Autodesk Inventor part; units mm, degrees
(part 6 of 6)
extrude "Zifferblatt" cut sketch "Text" against normal blind 1 contours S0 L450 S1 S2 L451 L452 L453 S3 S4 L454 L455 L456 S5 S6 L457 S7 L458 | S8 S9 S10 S11 L459 L460 S12 S13 S14 S15 L461 S16 S17 L462 | S18 S19 L463 S20 S21 L464 | S22 S23 L465 S24 S25 L466 | S26 S27 S28 S29 S30 L467 S31 S32 L468 S33 S34 L469 S35 S36 L470 S37 S38 S39 S40 S41 S42 L471 S43 S44 L472 S45 S46 S47 S48 S49 L473 S50 | S51 S52 S53 S54 S55 L474 S56 S57 S58 S59 S60 S61 S62 L475 S63 S64 | S65 S66 L476 L477 L478 S67 S68 L479 S69 S70 L480 L481 L482 S71 S72 L483 | S73 S74 L484 L485 S75 S76 S77 S78 L486 S79 S80 S81 S82 L487 S83 S84 S85 S86 L488 L489 L490 | S87 S88 L491 L492 S89 S90 L493 S91 L494 S92 S93 L495 L496 L497 | S94 S95 L498 S96 S97 L499 S98 S99 L500 S100 S101 L501 | S102 S103 S104 S105 | S106 S107 S108 S109 | S110 S111 L502 L503 S112 S113 L504 S114 L505 S115 S116 L506 L507 L508 | S117 S118 S119 S120 L509 L510 S121 S122 S123 S124 L511 S125 S126 S127 S128 L512 | S129 S130 L513 S131 S132 L514 | S133 L515 S134 S135 L516 L517 L518 S136 S137 L519 L520 L521 S138 S139 L522 S140 L523 | S141 S142 L524 S143 L525 L526 S144 S145 L527 S146 L528 S147 L529 S148 S149 L530 S150 S151 S152 S153 S154 S155 L531 S156 S157 S158 | S159 S160 L532 S161 S162 L533 L534 S163 S164 L535 L536 | S165 S166 L537 S167 S168 L538 S169 S170 L539 S171 S172 L540 | S173 S174 S175 S176 S177 S178 S179 L541 S180 S181 S182 S183 L542 S184 S185 S186 S187 L543 S188 S189 S190 S191 S192 S193 S194 L544 S195 S196 L545 | S197 S198 L546 S199 S200 L547 | S201 S202 L548 L549 S203 S204 L550 S205 L551 S206 S207 L552 L553 L554 | S208 S209 L555 S210 S211 L556 L557 S212 S213 L558 S214 S215 L559 L560 | S216 S217 L561 L562 S218 S219 S220 S221 L563 S222 S223 S224 S225 L564 S226 S227 S228 S229 L565 L566 L567 | S230 S231 S232 S233 | S234 S235 S236 S237 | S238 S239 L568 L569 S240 S241 S242 S243 L570 S244 S245 S246 S247 L571 S248 S249 S250 S251 L572 L573 L574 | S252 S253 S254 S255 | S256 S257 S258 S259 | S260 S261 L575 S262 L576 L577 S263 S264 L578 S265 L579 S266 L580 S267 S268 L581 S269 S270 S271 S272 S273 S274 L582 S275 S276 S277 | S278 S279 S280 S281 S282 S283 L583 S284 S285 S286 S287 S288 S289 S290 S291 L584 S292 S293 | S294 S295 S296 S297 S298 S299 L585 S300 S301 S302 S303 S304 S305 S306 S307 L586 S308 S309 | S310 S311 S312 S313 L587 L588 S314 S315 S316 S317 L589 S318 S319 S320 S321 L590 | S322 S323 L591 S324 S325 L592 | S326 S327 S328 S329 S330 L593 S331 S332 L594 S333 S334 L595 S335 S336 L596 S337 S338 S339 S340 S341 S342 L597 S343 S344 L598 S345 S346 S347 S348 S349 L599 S350 | S351 S352 S353 S354 S355 L600 S356 L601 L602 L603 S357 S358 L604 S359 L605 S360 L606 S361 L607 S362 S363 | S364 S365 L608 S366 S367 L609 L610 S368 S369 L611 S370 S371 L612 L613 | S372 S373 L614 S374 S375 S376 L615 L616 S377 S378 L617 S379 S380 S381 S382 L618 L619 | S383 S384 L620 L621 S385 S386 S387 S388 L622 S389 S390 S391 S392 L623 S393 S394 S395 S396 L624 L625 L626 | S397 S398 S399 S400 | S401 S402 S403 S404 | S405 S406 S407 S408 L627 L628 S409 S410 S411 S412 L629 S413 S414 S415 S416 L630 L631 S417 S418 L632 L633 S419 S420 S421 S422 L634 | S423 S424 L635 S425 S426 L636 L637 S427 S428 L638 S429 S430 L639 L640 | S431 S432 L641 L642 S433 S434 S435 S436 L643 S437 S438 S439 S440 L644 S441 S442 S443 S444 L645 L646 L647 | S445 S446 S447 S448 S449 S450 S451 L648 S452 S453 S454 S455 L649 S456 S457 S458 S459 L650 S460 S461 S462 S463 S464 S465 S466 L651 S467 S468 L652 | S469 S470 L653 S471 S472 L654 | S473 S474 S475 S476 S477 S478 L655 S479 S480 S481 S482 S483 S484 S485 S486 L656 S487 S488 | S489 S490 S491 S492 S493 S494 L657 S495 S496 S497 S498 S499 S500 S501 S502 L658 S503 S504 | S505 S506 L659 L660 L661 S507 S508 L662 S509 S510 L663 L664 L665 S511 S512 L666 | S513 S514 L667 L668 S515 S516 S517 S518 L669 S519 S520 S521 S522 L670 S523 S524 S525 S526 L671 L672 L673 | S527 S528 L674 S529 S530 L675 S531 S532 L676 S533 S534 L677 | S535 S536 S537 S538 S539 S540 S541 L678 S542 S543 S544 S545 L679 S546 S547 S548 S549 L680 S550 S551 S552 S553 S554 S555 S556 L681 S557 S558 L682 | S559 S560 L683 S561 S562 L684 | S563 S564 L685 S565 S566 L686 | S567 L687 S568 S569 L688 L689 L690 S570 S571 L691 L692 L693 S572 S573 L694 S574 L695 | S575 S576 S577 S578 S579 L696 S580 L697 L698 L699 S581 S582 L700 S583 L701 S584 L702 S585 L703 S586 S587 | S588 L704 S589 S590 L705 L706 L707 S591 S592 L708 L709 L710 S593 S594 L711 S595 L712 | S596 S597 S598 S599 L713 L714 S600 S601 S602 S603 L715 S604 S605 S606 S607 L716 | S608 S609 L717 S610 S611 L718 | S612 L719 S613 S614 L720 L721 L722 S615 S616 L723 L724 L725 S617 S618 L726 S619 L727 | S620 S621 L728 S622 L729 L730 S623 S624 L731 S625 L732 S626 L733 S627 S628 L734 S629 S630 S631 S632 S633 S634 L735 S635 S636 S637 | S638 S639 L736 S640 S641 L737 | S642 S643 L738 L739 S644 S645 L740 S646 L741 S647 S648 L742 L743 L744 | S649 S650 L745 S651 S652 L746 S653 S654 L747 S655 S656 L748 | S657 S658 S659 S660 | S661 S662 S663 S664 | S665 S666 L749 L750 S667 S668 L751 S669 L752 S670 S671 L753 L754 L755 | S672 S673 L756 S674 S675 L757 | S676 S677 S678 S679 S680 L758 S681 S682 L759 S683 L760 S684 S685 S686 S687 S688 S689 L761 S690 S691 L762 S692 S693 L763 S694 | S695 S696 L764 S697 S698 L765 L766 S699 S700 L767 L768 | S701 S702 S703 S704 S705 L769 S706 S707 L770 S708 S709 L771 S710 S711 L772 S712 S713 S714 S715 S716 S717 L773 S718 S719 L774 S720 S721 S722 S723 S724 L775 S725 | S726 S727 L776 L777 S728 S729 S730 S731 L778 S732 S733 S734 S735 L779 S736 S737 S738 S739 L780 L781 L782 | S740 S741 S742 S743 | S744 S745 S746 S747 | S748 S749 S750 S751 S752 L783 S753 S754 S755 S756 S757 S758 S759 L784 S760 S761 | S762 S763 L785 L786 L787 S764 S765 L788 S766 S767 L789 L790 L791 S768 S769 L792 | S770 S771 S772 S773 S774 L793 S775 S776 L794 S777 S778 L795 S779 S780 L796 S781 S782 S783 S784 S785 S786 L797 S787 S788 L798 S789 S790 S791 S792 S793 L799 S794 | S795 S796 L800 S797 S798 L801 | S799 S800 S801 S802 S803 L802 S804 S805 L803 S806 S807 L804 S808 S809 L805 S810 S811 S812 S813 S814 S815 L806 S816 S817 L807 S818 S819 S820 S821 S822 L808 S823 | S824 S825 L809 S826 S827 L810 | S828 S829 S830 S831 S832 S833 S834 L811 S835 S836 S837 S838 L812 S839 S840 S841 S842 L813 S843 S844 S845 S846 S847 S848 S849 L814 S850 S851 L815 | S852 S853 L816 S854 S855 L817 | S856 S857 L818 S858 S859 S860 L819 L820 S861 S862 L821 S863 S864 S865 S866 L822 L823 | S867 S868 L824 S869 S870 L825 | S871 S872 L826 L827 S873 S874 S875 S876 L828 S877 S878 S879 S880 L829 S881 S882 S883 S884 L830 L831 L832 | S885 S886 S887 S888 S889 L833 S890 S891 S892 S893 S894 S895 S896 L834 S897 S898 | S899 S900 L835 L836 L837 S901 S902 L838 S903 S904 L839 L840 L841 S905 S906 L842 | S907 S908 L843 S909 S910 L844 L845 S911 S912 L846 L847 | S913 S914 L848 S915 S916 L849 | S917 S918 L850 S919 S920 S921 L851 L852 S922 S923 L853 S924 S925 S926 S927 L854 L855 | S928 S929 L856 S930 S931 L857 S932 S933 L858 S934 S935 L859 | S936 S937 S938 S939 | S940 S941 S942 S943 | S944 S945 L860 S946 S947 S948 L861 L862 S949 S950 L863 S951 S952 S953 S954 L864 L865 | S955 S956 L866 S957 S958 L867 | S959 L868 S960 S961 L869 L870 L871 S962 S963 L872 L873 L874 S964 S965 L875 S966 L876 | S967 S968 L877 L878 S969 S970 L879 S971 L880 | S972 S973 L881 S974 S975 L882 L883 S976 S977 L884 S978 S979 L885 L886 | S980 S981 L887 L888 S982 S983 S984 S985 L889 S986 S987 S988 S989 L890 S990 S991 S992 S993 L891 L892 L893 | S994 S995 S996 S997 | S998 S999 S1000 S1001 | S1002 S1003 L894 S1004 S1005 S1006 L895 L896 S1007 S1008 L897 S1009 S1010 S1011 S1012 L898 L899 | S1013 S1014 L900 S1015 S1016 L901 | S1017 L902 S1018 S1019 L903 L904 L905 S1020 S1021 L906 L907 L908 S1022 S1023 L909 S1024 L910 | S1025 S1026 L911 S1027 L912 L913 S1028 S1029 L914 S1030 L915 S1031 L916 S1032 S1033 L917 S1034 S1035 S1036 S1037 S1038 S1039 L918 S1040 S1041 S1042 | S1043 S1044 S1045 S1046 S1047 S1048 S1049 L919 S1050 S1051 S1052 S1053 L920 S1054 S1055 S1056 S1057 L921 S1058 S1059 S1060 S1061 S1062 S1063 S1064 L922 S1065 S1066 L923 | S1067 S1068 L924 S1069 S1070 L925 | S1071 S1072 S1073 S1074 S1075 S1076 L926 S1077 S1078 S1079 S1080 S1081 S1082 S1083 S1084 L927 S1085 S1086 | S1087 S1088 S1089 S1090 S1091 S1092 L928 S1093 S1094 S1095 S1096 S1097 S1098 S1099 S1100 L929 S1101 S1102 | S1103 S1104 S1105 S1106 | S1107 S1108 S1109 S1110 | S1111 S1112 L930 S1113 S1114 L931 S1115 S1116 L932 S1117 S1118 L933 | S1119 S1120 L934 L935 S1121 S1122 L936 S1123 L937 S1124 S1125 L938 L939 L940 | S1126 S1127 L941 S1128 S1129 L942 | S1130 S1131 L943 S1132 S1133 L944 L945 S1134 S1135 L946 S1136 S1137 L947 L948 | S1138 S1139 S1140 S1141 L949 L950 S1142 S1143 S1144 S1145 L951 S1146 S1147 S1148 S1149 L952 L953 S1150 S1151 L954 L955 S1152 S1153 S1154 S1155 L956 | S1156 S1157 S1158 S1159 S1160 S1161 L957 S1162 S1163 S1164 S1165 S1166 S1167 S1168 S1169 L958 S1170 S1171 | S1172 S1173 S1174 S1175 S1176 S1177 L959 S1178 S1179 S1180 S1181 S1182 S1183 S1184 S1185 L960 S1186 S1187 | S1188 S1189 S1190 S1191 | S1192 S1193 S1194 S1195 | S1196 S1197 L961 S1198 S1199 L962 S1200 S1201 L963 S1202 S1203 L964 | S1204 S1205 L965 L966 S1206 S1207 L967 S1208 L968 S1209 S1210 L969 L970 L971 | S1211 S1212 L972 S1213 S1214 L973 | S1215 S1216 L974 S1217 S1218 S1219 L975 L976 S1220 S1221 L977 S1222 S1223 S1224 S1225 L978 L979 | S1226 S1227 L980 L981 S1228 S1229 S1230 S1231 L982 S1232 S1233 S1234 S1235 L983 S1236 S1237 S1238 S1239 L984 L985 L986 | S1240 S1241 L987 S1242 S1243 L988 S1244 S1245 L989 S1246 S1247 L990 | S1248 S1249 L991 L992 L993 S1250 S1251 L994 S1252 S1253 L995 L996 L997 S1254 S1255 L998 | S1256 S1257 L999 S1258 L1000 L1001 S1259 S1260 L1002 S1261 L1003 S1262 L1004 S1263 S1264 L1005 S1265 S1266 S1267 S1268 S1269 S1270 L1006 S1271 S1272 S1273 | S1274 S1275 S1276 S1277 S1278 L1007 S1279 S1280 L1008 S1281 S1282 L1009 S1283 S1284 L1010 S1285 S1286 S1287 S1288 S1289 S1290 L1011 S1291 S1292 L1012 S1293 S1294 S1295 S1296 S1297 L1013 S1298 | S1299 L1014 S1300 S1301 L1015 L1016 L1017 S1302 S1303 L1018 L1019 L1020 S1304 S1305 L1021 S1306 L1022 | S1307 S1308 L1023 S1309 S1310 L1024 | S1311 S1312 S1313 S1314 S1315 L1025 S1316 S1317 L1026 S1318 S1319 L1027 S1320 S1321 L1028 S1322 S1323 S1324 S1325 S1326 S1327 L1029 S1328 S1329 L1030 S1330 S1331 S1332 S1333 S1334 L1031 S1335 | S1336 S1337 L1032 S1338 S1339 L1033 L1034 S1340 S1341 L1035 S1342 S1343 L1036 L1037 | S1344 S1345 S1346 S1347 L1038 L1039 S1348 S1349 S1350 S1351 L1040 S1352 S1353 S1354 S1355 L1041 L1042 S1356 S1357 L1043 L1044 S1358 S1359 S1360 S1361 L1045 | S1362 S1363 S1364 S1365 S1366 S1367 L1046 S1368 S1369 S1370 S1371 S1372 S1373 S1374 S1375 L1047 S1376 S1377 | S1378 S1379 S1380 S1381 S1382 S1383 L1048 S1384 S1385 S1386 S1387 S1388 S1389 S1390 S1391 L1049 S1392 S1393 | S1394 S1395 S1396 S1397 | S1398 S1399 S1400 S1401 | S1402 S1403 L1050 S1404 S1405 L1051 | S1406 S1407 S1408 S1409 S1410 L1052 S1411 S1412 L1053 S1413 S1414 L1054 S1415 S1416 L1055 S1417 S1418 S1419 S1420 S1421 S1422 L1056 S1423 S1424 L1057 S1425 S1426 S1427 S1428 S1429 L1058 S1430 | S1431 S1432 L1059 S1433 L1060 L1061 S1434 S1435 L1062 S1436 L1063 S1437 L1064 S1438 S1439 S1440 S1441 S1442 | S1443 S1444 L1065 S1445 L1066 L1067 S1446 S1447 L1068 S1448 L1069 S1449 L1070 S1450 S1451 L1071 S1452 S1453 S1454 S1455 S1456 S1457 L1072 S1458 S1459 S1460 | S1461 S1462 L1073 S1463 S1464 L1074 S1465 S1466 L1075 S1467 S1468 L1076 | S1469 S1470 S1471 S1472 | S1473 S1474 S1475 S1476
sketch "Skizze5" plane through (0, 0, 0) normal (0, 0, -1) x (-1, 0, 0)
  line L0 (-16.665, 0) -> (16.665, 0)
  line L1 (16.665, 0) -> (16.665, -36)
  line L2 (16.665, -36) -> (-16.665, -36)
  line L3 (-16.665, -36) -> (-16.665, 0)
  line L4 (16.665, -36) -> (16.665, 0)
  line L5 (16.665, 0) -> (49.995, 0)
  line L6 (49.995, 0) -> (49.995, -36)
  line L7 (49.995, -36) -> (16.665, -36)
  line L8 (49.995, -36) -> (49.995, 0)
  line L9 (49.995, 0) -> (83.325, 0)
  line L10 (83.325, 0) -> (83.325, -36)
  line L11 (83.325, -36) -> (49.995, -36)
  line L12 (83.325, -36) -> (83.325, 0)
  line L13 (83.325, 0) -> (116.655, 0)
  line L14 (116.655, 0) -> (116.655, -36)
  line L15 (116.655, -36) -> (83.325, -36)
  line L16 (116.655, -36) -> (116.655, 0)
  line L17 (116.655, 0) -> (149.985, 0)
  line L18 (149.985, 0) -> (149.985, -36)
  line L19 (149.985, -36) -> (116.655, -36)
  line L20 (149.985, -36) -> (149.985, 0)
  line L21 (149.985, 0) -> (183.315, 0)
  line L22 (183.315, 0) -> (183.315, -36)
  line L23 (183.315, -36) -> (149.985, -36)
  line L24 (183.315, -36) -> (183.315, 0)
  line L25 (183.315, 0) -> (216.645, 0)
  line L26 (216.645, 0) -> (216.645, -36)
  line L27 (216.645, -36) -> (183.315, -36)
  line L28 (-16.665, 0) -> (-16.665, 36)
  line L29 (-16.665, 36) -> (16.665, 36)
  line L30 (16.665, 36) -> (16.665, 0)
  line L31 (16.665, 0) -> (-16.665, 0)
  line L32 (16.665, 0) -> (16.665, 36)
  line L33 (16.665, 36) -> (49.995, 36)
  line L34 (49.995, 36) -> (49.995, 0)
  line L35 (49.995, 0) -> (16.665, 0)
  line L36 (49.995, 0) -> (49.995, 36)
  line L37 (49.995, 36) -> (83.325, 36)
  line L38 (83.325, 36) -> (83.325, 0)
  line L39 (83.325, 0) -> (49.995, 0)
  line L40 (83.325, 0) -> (83.325, 36)
  line L41 (83.325, 36) -> (116.655, 36)
  line L42 (116.655, 36) -> (116.655, 0)
  line L43 (116.655, 0) -> (83.325, 0)
  line L44 (116.655, 0) -> (116.655, 36)
  line L45 (116.655, 36) -> (149.985, 36)
  line L46 (149.985, 36) -> (149.985, 0)
  line L47 (149.985, 0) -> (116.655, 0)
  line L48 (149.985, 0) -> (149.985, 36)
  line L49 (149.985, 36) -> (183.315, 36)
  line L50 (183.315, 36) -> (183.315, 0)
  line L51 (183.315, 0) -> (149.985, 0)
  line L52 (183.315, 0) -> (183.315, 36)
  line L53 (183.315, 36) -> (216.645, 36)
  line L54 (216.645, 36) -> (216.645, 0)
  line L55 (216.645, 0) -> (183.315, 0)
  line L56 (-16.665, 36) -> (-16.665, 72)
  line L57 (-16.665, 72) -> (16.665, 72)
  line L58 (16.665, 72) -> (16.665, 36)
  line L59 (16.665, 36) -> (-16.665, 36)
  line L60 (16.665, 36) -> (16.665, 72)
  line L61 (16.665, 72) -> (49.995, 72)
  line L62 (49.995, 72) -> (49.995, 36)
  line L63 (49.995, 36) -> (16.665, 36)
  line L64 (49.995, 36) -> (49.995, 72)
  line L65 (49.995, 72) -> (83.325, 72)
  line L66 (83.325, 72) -> (83.325, 36)
  line L67 (83.325, 36) -> (49.995, 36)
  line L68 (83.325, 36) -> (83.325, 72)
  line L69 (83.325, 72) -> (116.655, 72)
  line L70 (116.655, 72) -> (116.655, 36)
  line L71 (116.655, 36) -> (83.325, 36)
  line L72 (116.655, 36) -> (116.655, 72)
  line L73 (116.655, 72) -> (149.985, 72)
  line L74 (149.985, 72) -> (149.985, 36)
  line L75 (149.985, 36) -> (116.655, 36)
  line L76 (149.985, 36) -> (149.985, 72)
  line L77 (149.985, 72) -> (183.315, 72)
  line L78 (183.315, 72) -> (183.315, 36)
  line L79 (183.315, 36) -> (149.985, 36)
  line L80 (183.315, 36) -> (183.315, 72)
  line L81 (183.315, 72) -> (216.645, 72)
  line L82 (216.645, 72) -> (216.645, 36)
  line L83 (216.645, 36) -> (183.315, 36)
  line L84 (-16.665, 72) -> (-16.665, 108)
  line L85 (-16.665, 108) -> (16.665, 108)
  line L86 (16.665, 108) -> (16.665, 72)
  line L87 (16.665, 72) -> (-16.665, 72)
  line L88 (16.665, 72) -> (16.665, 108)
  line L89 (16.665, 108) -> (49.995, 108)
  line L90 (49.995, 108) -> (49.995, 72)
  line L91 (49.995, 72) -> (16.665, 72)
  line L92 (49.995, 72) -> (49.995, 108)
  line L93 (49.995, 108) -> (83.325, 108)
  line L94 (83.325, 108) -> (83.325, 72)
  line L95 (83.325, 72) -> (49.995, 72)
  line L96 (83.325, 72) -> (83.325, 108)
  line L97 (83.325, 108) -> (116.655, 108)
  line L98 (116.655, 108) -> (116.655, 72)
  line L99 (116.655, 72) -> (83.325, 72)
  line L100 (116.655, 72) -> (116.655, 108)
  line L101 (116.655, 108) -> (149.985, 108)
  line L102 (149.985, 108) -> (149.985, 72)
  line L103 (149.985, 72) -> (116.655, 72)
  line L104 (149.985, 72) -> (149.985, 108)
  line L105 (149.985, 108) -> (183.315, 108)
  line L106 (183.315, 108) -> (183.315, 72)
  line L107 (183.315, 72) -> (149.985, 72)
  line L108 (183.315, 72) -> (183.315, 108)
  line L109 (183.315, 108) -> (216.645, 108)
  line L110 (216.645, 108) -> (216.645, 72)
  line L111 (216.645, 72) -> (183.315, 72)
  line L112 (-16.665, 108) -> (-16.665, 144)
  line L113 (-16.665, 144) -> (16.665, 144)
  line L114 (16.665, 144) -> (16.665, 108)
  line L115 (16.665, 108) -> (-16.665, 108)
  line L116 (16.665, 108) -> (16.665, 144)
  line L117 (16.665, 144) -> (49.995, 144)
  line L118 (49.995, 144) -> (49.995, 108)
  line L119 (49.995, 108) -> (16.665, 108)
  line L120 (49.995, 108) -> (49.995, 144)
  line L121 (49.995, 144) -> (83.325, 144)
  line L122 (83.325, 144) -> (83.325, 108)
  line L123 (83.325, 108) -> (49.995, 108)
  line L124 (83.325, 108) -> (83.325, 144)
  line L125 (83.325, 144) -> (116.655, 144)
  line L126 (116.655, 144) -> (116.655, 108)
  line L127 (116.655, 108) -> (83.325, 108)
  line L128 (116.655, 108) -> (116.655, 144)
  line L129 (116.655, 144) -> (149.985, 144)
  line L130 (149.985, 144) -> (149.985, 108)
  line L131 (149.985, 108) -> (116.655, 108)
  line L132 (149.985, 108) -> (149.985, 144)
  line L133 (149.985, 144) -> (183.315, 144)
  line L134 (183.315, 144) -> (183.315, 108)
  line L135 (183.315, 108) -> (149.985, 108)
  line L136 (183.315, 108) -> (183.315, 144)
  line L137 (183.315, 144) -> (216.645, 144)
  line L138 (216.645, 144) -> (216.645, 108)
  line L139 (216.645, 108) -> (183.315, 108)
  line L140 (-16.665, 144) -> (-16.665, 180)
  line L141 (-16.665, 180) -> (16.665, 180)
  line L142 (16.665, 180) -> (16.665, 144)
  line L143 (16.665, 144) -> (-16.665, 144)
  line L144 (16.665, 144) -> (16.665, 180)
  line L145 (16.665, 180) -> (49.995, 180)
  line L146 (49.995, 180) -> (49.995, 144)
  line L147 (49.995, 144) -> (16.665, 144)
  line L148 (49.995, 144) -> (49.995, 180)
  line L149 (49.995, 180) -> (83.325, 180)
  line L150 (83.325, 180) -> (83.325, 144)
  line L151 (83.325, 144) -> (49.995, 144)
  line L152 (83.325, 144) -> (83.325, 180)
  line L153 (83.325, 180) -> (116.655, 180)
  line L154 (116.655, 180) -> (116.655, 144)
  line L155 (116.655, 144) -> (83.325, 144)
  line L156 (116.655, 144) -> (116.655, 180)
  line L157 (116.655, 180) -> (149.985, 180)
  line L158 (149.985, 180) -> (149.985, 144)
  line L159 (149.985, 144) -> (116.655, 144)
  line L160 (149.985, 144) -> (149.985, 180)
  line L161 (149.985, 180) -> (183.315, 180)
  line L162 (183.315, 180) -> (183.315, 144)
  line L163 (183.315, 144) -> (149.985, 144)
  line L164 (183.315, 144) -> (183.315, 180)
  line L165 (183.315, 180) -> (216.645, 180)
  line L166 (216.645, 180) -> (216.645, 144)
  line L167 (216.645, 144) -> (183.315, 144)
  line L168 (-16.665, 180) -> (-16.665, 216)
  line L169 (-16.665, 216) -> (16.665, 216)
  line L170 (16.665, 216) -> (16.665, 180)
  line L171 (16.665, 180) -> (-16.665, 180)
  line L172 (16.665, 180) -> (16.665, 216)
  line L173 (16.665, 216) -> (49.995, 216)
  line L174 (49.995, 216) -> (49.995, 180)
  line L175 (49.995, 180) -> (16.665, 180)
  line L176 (49.995, 180) -> (49.995, 216)
  line L177 (49.995, 216) -> (83.325, 216)
  line L178 (83.325, 216) -> (83.325, 180)
  line L179 (83.325, 180) -> (49.995, 180)
  line L180 (83.325, 180) -> (83.325, 216)
  line L181 (83.325, 216) -> (116.655, 216)
  line L182 (116.655, 216) -> (116.655, 180)
  line L183 (116.655, 180) -> (83.325, 180)
  line L184 (116.655, 180) -> (116.655, 216)
  line L185 (116.655, 216) -> (149.985, 216)
  line L186 (149.985, 216) -> (149.985, 180)
  line L187 (149.985, 180) -> (116.655, 180)
  line L188 (149.985, 180) -> (149.985, 216)
  line L189 (149.985, 216) -> (183.315, 216)
  line L190 (183.315, 216) -> (183.315, 180)
  line L191 (183.315, 180) -> (149.985, 180)
  line L192 (183.315, 180) -> (183.315, 216)
  line L193 (183.315, 216) -> (216.645, 216)
  line L194 (216.645, 216) -> (216.645, 180)
  line L195 (216.645, 180) -> (183.315, 180)
  line L196 (230, -230) -> (230, 230) projected
  line L197 (230, 230) -> (-230, 230) projected
  line L198 (-216.645, 210.8033) -> (-185.6407, 210.8033)
  line L199 (-185.6407, 210.8033) -> (-185.6407, 180)
  line L200 (-185.6407, 180) -> (-216.645, 180)
  line L201 (-216.645, 180) -> (-216.645, 210.8033)
  line L202 (-230, 230) -> (-230, -230) projected
  line L203 (216.645, -216) -> (183.315, -216)
  line L204 (183.315, -216) -> (183.315, -182.4848)
  line L205 (183.315, -182.4848) -> (216.645, -182.4848)
  line L206 (216.645, -182.4848) -> (216.645, -216)
  line L207 (-230, -230) -> (230, -230) projected
  point P0 (0, 0)
  point P1 (0, 0)
  point P2 (33.33, 0)
  point P3 (66.66, 0)
  point P4 (99.99, 0)
  point P5 (133.32, 0)
  point P6 (166.65, 0)
  point P7 (199.98, 0)
  point P8 (0, 36)
  point P9 (33.33, 36)
  point P10 (66.66, 36)
  point P11 (99.99, 36)
  point P12 (133.32, 36)
  point P13 (166.65, 36)
  point P14 (199.98, 36)
  point P15 (0, 72)
  point P16 (33.33, 72)
  point P17 (66.66, 72)
  point P18 (99.99, 72)
  point P19 (133.32, 72)
  point P20 (166.65, 72)
  point P21 (199.98, 72)
  point P22 (0, 108)
  point P23 (33.33, 108)
  point P24 (66.66, 108)
  point P25 (99.99, 108)
  point P26 (133.32, 108)
  point P27 (166.65, 108)
  point P28 (199.98, 108)
  point P29 (0, 144)
  point P30 (33.33, 144)
  point P31 (66.66, 144)
  point P32 (99.99, 144)
  point P33 (133.32, 144)
  point P34 (166.65, 144)
  point P35 (199.98, 144)
  point P36 (0, 180)
  point P37 (33.33, 180)
  point P38 (66.66, 180)
  point P39 (99.99, 180)
  point P40 (133.32, 180)
  point P41 (166.65, 180)
  point P42 (199.98, 180)
  point P43 (0, 216)
  point P44 (33.33, 216)
  point P45 (66.66, 216)
  point P46 (99.99, 216)
  point P47 (133.32, 216)
  point P48 (166.65, 216)
  point P49 (199.98, 216)
  point P50 (199.98, 198)
  point P51 (166.65, 198)
  point P52 (199.98, 216)
  point P53 (166.65, 216)
  point P54 (149.985, 198)
  dimension "d153" = 36
  dimension "d154" = 33.33
  dimension "d157" = 33.33
  dimension "d160" = 36
  dimension "d166" = 14
  dimension "d167" = 36
  dimension "d168" = 33.33
  dimension "d169" = 13.355
  dimension "d170" = 13.355
  dimension "d171" = 433.29
  dimension "d172" = 46.685
  dimension "d173" = 446.645
  dimension "d174" = 50
  dimension "d175" = 14
  dimension "d176" = 446
  constraints: 408 end point, 6 parallel, 4 horizontal, 4 midpoint, 3 perpendicular, 2 collinear, 2 horizontal alignment, 2 vertical alignment, 1 coincident, 1 vertical, 430 other
  measures "d153" distance of L0.end L1.end
  measures "d154" distance of L1.end L2.end
  measures "d157" distance of L2.end L4.start
  measures "d160" distance of L2.end L28.start
  measures "d166" distance between parallel lines of L197 L193
  measures "d167" distance between parallel lines of L195 L193
  measures "d168" distance between parallel lines of L190 L194
  measures "d169" distance between parallel lines of L196 L194
  measures "d170" distance between parallel lines of L201 L202
  measures "d171" distance between parallel lines of L201 L194
  measures "d172" distance between parallel lines of L190 L196
  measures "d173" distance between parallel lines of L201 L196
  measures "d174" distance between parallel lines of L165 L197
  measures "d175" distance between parallel lines of L207 L203
  measures "d176" distance between parallel lines of L203 L197
equation "\"d36\" = Aussenmass"
equation "\"d43\" = 0.913043 * Aussenmass"
equation "\"d83\" = 0.5 * Teilung"
equation "\"d106\" = Teilung"
equation "\"Teilung\" = 33.33333"
equation "\"Aussenmass\" = 460"
